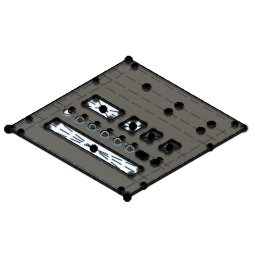
nts-1 v14 (Autodesk Fusion 360 design; units mm, degrees)
Autodesk Fusion 360 part; units mm, degrees
sketch "Sketch1" plane through (0, 0, 0) normal (0, 0, 1) x (1, 0, 0)
  line L0 (2, 0) -> (126.53, 0)
  line L1 (128.53, 2) -> (128.53, 128)
  line L2 (126.53, 130) -> (2, 130)
  line L3 (0, 128) -> (0, 2)
  line L4 (0, 70) -> (128.53, 70) construction
  line L5 (0, 46.94) -> (128.53, 46.94) construction
  line L6 (0, 92) -> (128.53, 92) construction
  line L7 (0, 20) -> (128.53, 20) construction
  line L8 (2.5, 130) -> (2.5, 0) construction
  line L9 (126.03, 130) -> (126.03, 0) construction
  circle A0 centre (71, 46.94) radius 3.55
  circle A1 centre (17, 46.94) radius 3.55
  circle A2 centre (84.5, 46.94) radius 3.55
  circle A3 centre (30.5, 46.94) radius 3.55
  circle A4 centre (111.53, 46.94) radius 3.55
  circle A5 centre (44, 46.94) radius 3.55
  circle A6 centre (57.5, 46.94) radius 3.55
  circle A7 centre (126.03, 92) radius 1.5
  circle A8 centre (2.5, 92) radius 1.5
  circle A9 centre (2.5, 20) radius 1.5
  circle A10 centre (126.03, 20) radius 1.5
  line L10 (107.73, 62.5) -> (101.33, 62.5)
  line L11 (99.03, 64.8) -> (99.03, 75.2)
  line L12 (101.33, 77.5) -> (107.73, 77.5)
  line L13 (110.03, 75.2) -> (110.03, 64.8)
  line L14 (110.03, 62.5) -> (99.03, 77.5) construction
  line L15 (99.03, 62.5) -> (110.03, 77.5) construction
  line L16 (88.03, 62.5) -> (81.33, 62.5)
  line L17 (79.03, 64.8) -> (79.03, 75.5)
  line L18 (81.03, 77.5) -> (88.03, 77.5)
  line L19 (90.03, 75.5) -> (90.03, 64.5)
  line L20 (90.03, 62.5) -> (79.03, 77.5) construction
  line L21 (79.03, 62.5) -> (90.03, 77.5) construction
  line L22 (70.03, 61.5) -> (59.03, 61.5)
  line L23 (57.03, 63.5) -> (57.03, 76.5)
  line L24 (59.03, 78.5) -> (70.03, 78.5)
  line L25 (72.03, 76.5) -> (72.03, 63.5)
  line L26 (72.03, 61.5) -> (57.03, 78.5) construction
  line L27 (57.03, 61.5) -> (72.03, 78.5) construction
  line L28 (46.53, 62) -> (18.53, 62)
  line L29 (16.53, 64) -> (16.53, 76)
  line L30 (18.53, 78) -> (46.53, 78)
  line L31 (48.53, 76) -> (48.53, 64)
  line L32 (48.53, 62) -> (16.53, 78) construction
  line L33 (16.53, 62) -> (48.53, 78) construction
  line L34 (100.23, 49.94) -> (94.83, 49.94)
  line L35 (92.53, 47.64) -> (92.53, 46.24)
  line L36 (94.83, 43.94) -> (100.23, 43.94)
  line L37 (102.53, 46.24) -> (102.53, 47.64)
  line L38 (102.53, 49.94) -> (92.53, 43.94) construction
  line L39 (92.53, 49.94) -> (102.53, 43.94) construction
  arc A11 (2, 130) -> (0, 128) centre (2, 128) ccw
  arc A12 (128.53, 128) -> (126.53, 130) centre (126.53, 128) ccw
  arc A13 (126.53, 0) -> (128.53, 2) centre (126.53, 2) ccw
  arc A14 (0, 2) -> (2, 0) centre (2, 2) ccw
  arc A15 (18.53, 78) -> (16.53, 76) centre (18.53, 76) ccw
  arc A16 (46.53, 62) -> (48.53, 64) centre (46.53, 64) ccw
  arc A17 (16.53, 64) -> (18.53, 62) centre (18.53, 64) ccw
  arc A18 (48.53, 76) -> (46.53, 78) centre (46.53, 76) ccw
  arc A19 (59.03, 78.5) -> (57.03, 76.5) centre (59.03, 76.5) ccw
  arc A20 (72.03, 76.5) -> (70.03, 78.5) centre (70.03, 76.5) ccw
  arc A21 (70.03, 61.5) -> (72.03, 63.5) centre (70.03, 63.5) ccw
  arc A22 (57.03, 63.5) -> (59.03, 61.5) centre (59.03, 63.5) ccw
  arc A23 (81.03, 77.5) -> (79.03, 75.5) centre (81.03, 75.5) ccw
  arc A24 (90.03, 75.5) -> (88.03, 77.5) centre (88.03, 75.5) ccw
  arc A25 (88.03, 62.5) -> (90.03, 64.5) centre (88.03, 64.5) ccw
  arc A26 (79.03, 64.8) -> (81.33, 62.5) centre (81.33, 64.8) ccw
  arc A27 (101.33, 77.5) -> (99.03, 75.2) centre (101.33, 75.2) ccw
  arc A28 (110.03, 75.2) -> (107.73, 77.5) centre (107.73, 75.2) ccw
  arc A29 (107.73, 62.5) -> (110.03, 64.8) centre (107.73, 64.8) ccw
  arc A30 (99.03, 64.8) -> (101.33, 62.5) centre (101.33, 64.8) ccw
  arc A31 (94.83, 49.94) -> (92.53, 47.64) centre (94.83, 47.64) ccw
  arc A32 (102.53, 47.64) -> (100.23, 49.94) centre (100.23, 47.64) ccw
  arc A33 (92.53, 46.24) -> (94.83, 43.94) centre (94.83, 46.24) ccw
  arc A34 (100.23, 43.94) -> (102.53, 46.24) centre (100.23, 46.24) ccw
  line L40 (0, 126.5) -> (128.53, 126.5) construction
  line L41 (0, 3.5) -> (128.53, 3.5) construction
  line L42 (118.53, 130) -> (118.53, 0) construction
  line L43 (10, 130) -> (10, 0) construction
  circle A35 centre (10, 126.5) radius 2
  circle A36 centre (118.53, 126.5) radius 2
  circle A37 centre (10, 3.5) radius 2
  circle A38 centre (118.53, 3.5) radius 2
  line L44 (0, 28) -> (128.53, 28) construction
  line L45 (109.765, 20.75) -> (18.765, 20.75)
  line L46 (16.765, 22.75) -> (16.765, 33.25)
  line L47 (18.765, 35.25) -> (109.765, 35.25)
  line L48 (111.765, 33.25) -> (111.765, 22.75)
  line L49 (111.765, 20.75) -> (16.765, 35.25) construction
  line L50 (16.765, 20.75) -> (111.765, 35.25) construction
  arc A39 (18.765, 35.25) -> (16.765, 33.25) centre (18.765, 33.25) ccw
  arc A40 (111.765, 33.25) -> (109.765, 35.25) centre (109.765, 33.25) ccw
  arc A41 (16.765, 22.75) -> (18.765, 20.75) centre (18.765, 22.75) ccw
  arc A42 (109.765, 20.75) -> (111.765, 22.75) centre (109.765, 22.75) ccw
  line L51 (0, 113.5) -> (128.53, 113.5) construction
  line L52 (0, 102) -> (128.53, 102) construction
  circle A43 centre (106.03, 113.5) radius 3.25
  circle A44 centre (106.03, 102) radius 3.25
  circle A45 centre (71.03, 113.5) radius 3.25
  circle A46 centre (71.03, 102) radius 3.25
  circle A47 centre (36.03, 113.5) radius 3.25
  line L53 (0, 51.84) -> (128.53, 51.84) construction
  circle A48 centre (17, 51.84) radius 0.75
  circle A49 centre (30.5, 51.84) radius 0.75
  circle A50 centre (44, 51.84) radius 0.75
  circle A51 centre (57.5, 51.84) radius 0.75
  circle A52 centre (71, 51.84) radius 0.75
  circle A53 centre (84.5, 51.84) radius 0.75
  circle A54 centre (111.53, 51.84) radius 0.75
  point P0 (128.53, 0)
  point P1 (0, 130)
  point P2 (104.53, 70)
  point P3 (84.53, 70)
  point P4 (64.53, 70)
  point P5 (32.53, 70)
  point P6 (97.53, 46.94)
  point P7 (64.265, 28)
  dimension "d1" = 128.53
  dimension "d2" = 130
  dimension "d4" = 2.5
  dimension "d5" = 2.5
  dimension "d7" = 60
  dimension "d25" = 7.1
  dimension "d26" = 7.1
  dimension "d27" = 7.1
  dimension "d28" = 7.1
  dimension "d29" = 7.1
  dimension "d30" = 7.1
  dimension "d31" = 7.1
  dimension "d32" = 17
  dimension "d33" = 13.5
  dimension "d34" = 13.5
  dimension "d35" = 13.5
  dimension "d36" = 13.5
  dimension "d37" = 13.5
  dimension "d38" = 17
  dimension "d42" = 3
  dimension "d43" = 3
  dimension "d44" = 3
  dimension "d45" = 3
  dimension "d49" = 72
  dimension "d54" = 23.06
  dimension "d55" = 22
  dimension "d56" = 11
  dimension "d57" = 15
  dimension "d58" = 24
  dimension "d59" = 11
  dimension "d60" = 15
  dimension "d61" = 20
  dimension "d62" = 15
  dimension "d63" = 17
  dimension "d64" = 20
  dimension "d65" = 32
  dimension "d66" = 16
  dimension "d67" = 32
  dimension "d68" = 10
  dimension "d69" = 6
  dimension "d70" = 14
  dimension "d75" = 2
  dimension "d76" = 2
  dimension "d77" = 2
  dimension "d78" = 2
  dimension "d79" = 2
  dimension "d80" = 2
  dimension "d81" = 2
  dimension "d82" = 2
  dimension "d83" = 2
  dimension "d84" = 2
  dimension "d85" = 2.3
  dimension "d86" = 123
  dimension "d87" = 3.5
  dimension "d89" = 4
  dimension "d90" = 4
  dimension "d91" = 4
  dimension "d92" = 4
  dimension "d93" = 10
  dimension "d94" = 10
  dimension "d99" = 42
  dimension "d100" = 95
  dimension "d101" = 14.5
  dimension "d102" = 2
  dimension "d103" = 2
  dimension "d104" = 2
  dimension "d105" = 2
  dimension "d106" = 32
  dimension "d107" = 11.5
  dimension "d110" = 6.5
  dimension "d111" = 6.5
  dimension "d112" = 6.5
  dimension "d113" = 6.5
  dimension "d117" = 35
  dimension "d118" = 20
  dimension "d121" = 6.5
  dimension "d122" = 35
  dimension "d123" = 4.9
  dimension "d126" = 1.5
  dimension "d127" = 17
  dimension "d128" = 1.5
  dimension "d129" = 1.5
  dimension "d130" = 1.5
  dimension "d131" = 1.5
  dimension "d132" = 1.5
  dimension "d133" = 1.5
  dimension "d134" = 17
  dimension "d135" = 13.5
  dimension "d136" = 13.5
  dimension "d137" = 13.5
  dimension "d138" = 13.5
  dimension "d139" = 13.5
  constraint horizontal L0
  constraint vertical L1
  constraint horizontal L2
  constraint vertical L3
  constraint coincident L3 L4.start
  constraint coincident L1 L4.end
  constraint perpendicular L1 L4
  constraint coincident L3 L5.start
  constraint perpendicular L3 L5
  constraint coincident L1 L5.end
  constraint coincident L3 L6.start
  constraint perpendicular L3 L6
  constraint coincident L1 L6.end
  constraint coincident L3 L7.start
  constraint perpendicular L3 L7
  constraint coincident L1 L7.end
  constraint coincident L2 L8.start
  constraint perpendicular L2 L8
  constraint coincident L0 L8.end
  constraint coincident L2 L9.start
  constraint perpendicular L2 L9
  constraint coincident L0 L9.end
  constraint coincident L5 A0.centre
  constraint coincident L5 A2.centre
  constraint coincident L5 A3.centre
  constraint coincident L5 A4.centre
  constraint coincident L5 A5.centre
  constraint coincident L5 A6.centre
  constraint coincident L9 A7.centre
  constraint coincident L6 A7.centre
  constraint coincident L8 A8.centre
  constraint coincident L6 A8.centre
  constraint coincident L8 A9.centre
  constraint coincident L7 A9.centre
  constraint coincident L9 A10.centre
  constraint coincident L7 A10.centre
  constraint horizontal L10
  constraint perpendicular L10 L11
  constraint parallel L10 L12
  constraint parallel L11 L13
  constraint coincident L14 P2
  constraint coincident L15 P2
  constraint coincident L4 P2
  constraint horizontal L16
  constraint perpendicular L16 L17
  constraint parallel L16 L18
  constraint parallel L17 L19
  constraint coincident L20 P3
  constraint coincident L21 P3
  constraint coincident L4 P3
  constraint horizontal L22
  constraint perpendicular L22 L23
  constraint parallel L22 L24
  constraint parallel L23 L25
  constraint coincident L26 P4
  constraint coincident L27 P4
  constraint coincident L4 P4
  constraint horizontal L28
  constraint perpendicular L28 L29
  constraint parallel L28 L30
  constraint parallel L29 L31
  constraint coincident L32 P5
  constraint coincident L33 P5
  constraint coincident L4 P5
  constraint horizontal L34
  constraint perpendicular L34 L35
  constraint parallel L34 L36
  constraint parallel L35 L37
  constraint coincident L38 P6
  constraint coincident L39 P6
  constraint coincident L5 P6
  constraint coincident P1 L2
  constraint coincident P1 L3
  constraint tangent L2 A11
  constraint tangent L3 A11
  constraint tangent L1 A12
  constraint tangent L2 A12
  constraint coincident P0 L0
  constraint coincident P0 L1
  constraint tangent L0 A13
  constraint tangent L1 A13
  constraint coincident origin L0
  constraint coincident origin L3
  constraint tangent L0 A14
  constraint tangent L3 A14
  constraint coincident L32.end L29
  constraint coincident L32.end L30
  constraint tangent L29 A15
  constraint tangent L30 A15
  constraint coincident L32.start L28
  constraint coincident L32.start L31
  constraint tangent L28 A16
  constraint tangent L31 A16
  constraint coincident L33.start L29
  constraint coincident L33.start L28
  constraint tangent L29 A17
  constraint tangent L28 A17
  constraint coincident L33.end L30
  constraint coincident L33.end L31
  constraint tangent L30 A18
  constraint tangent L31 A18
  constraint coincident L26.end L23
  constraint coincident L26.end L24
  constraint tangent L23 A19
  constraint tangent L24 A19
  constraint coincident L27.end L24
  constraint coincident L27.end L25
  constraint tangent L24 A20
  constraint tangent L25 A20
  constraint equal A19 A20
  constraint coincident L26.start L25
  constraint coincident L26.start L22
  constraint tangent L25 A21
  constraint tangent L22 A21
  constraint equal A19 A21
  constraint coincident L27.start L22
  constraint coincident L27.start L23
  constraint tangent L22 A22
  constraint tangent L23 A22
  constraint equal A19 A22
  constraint coincident L20.end L17
  constraint coincident L20.end L18
  constraint tangent L17 A23
  constraint tangent L18 A23
  constraint equal A19 A23
  constraint coincident L21.end L18
  constraint coincident L21.end L19
  constraint tangent L18 A24
  constraint tangent L19 A24
  constraint equal A19 A24
  constraint coincident L20.start L19
  constraint coincident L20.start L16
  constraint tangent L19 A25
  constraint tangent L16 A25
  constraint coincident L21.start L17
  constraint coincident L21.start L16
  constraint tangent L17 A26
  constraint tangent L16 A26
  constraint coincident L14.end L11
  constraint coincident L14.end L12
  constraint tangent L11 A27
  constraint tangent L12 A27
  constraint equal A26 A27
  constraint coincident L15.end L12
  constraint coincident L15.end L13
  constraint tangent L12 A28
  constraint tangent L13 A28
  constraint equal A26 A28
  constraint coincident L14.start L13
  constraint coincident L14.start L10
  constraint tangent L13 A29
  constraint tangent L10 A29
  constraint equal A26 A29
  constraint coincident L15.start L11
  constraint coincident L15.start L10
  constraint tangent L11 A30
  constraint tangent L10 A30
  constraint equal A26 A30
  constraint coincident L39.start L34
  constraint coincident L39.start L35
  constraint tangent L34 A31
  constraint tangent L35 A31
  constraint equal A26 A31
  constraint coincident L38.start L34
  constraint coincident L38.start L37
  constraint tangent L34 A32
  constraint tangent L37 A32
  constraint equal A26 A32
  constraint coincident L38.end L35
  constraint coincident L38.end L36
  constraint tangent L35 A33
  constraint tangent L36 A33
  constraint equal A26 A33
  constraint coincident L39.end L36
  constraint coincident L39.end L37
  constraint tangent L36 A34
  constraint tangent L37 A34
  constraint equal A26 A34
  constraint coincident L3 L40.start
  constraint perpendicular L3 L40
  constraint coincident L1 L40.end
  constraint coincident L3 L41.start
  constraint perpendicular L3 L41
  constraint coincident L1 L41.end
  constraint coincident L2 L42.start
  constraint coincident L0 L42.end
  constraint perpendicular L0 L42
  constraint coincident L2 L43.start
  constraint coincident L0 L43.end
  constraint perpendicular L0 L43
  constraint coincident L43 A35.centre
  constraint coincident L40 A35.centre
  constraint coincident L42 A36.centre
  constraint coincident L40 A36.centre
  constraint coincident L43 A37.centre
  constraint coincident L41 A37.centre
  constraint coincident L42 A38.centre
  constraint coincident L41 A38.centre
  constraint coincident L3 L44.start
  constraint perpendicular L3 L44
  constraint coincident L1 L44.end
  constraint horizontal L45
  constraint perpendicular L45 L46
  constraint parallel L45 L47
  constraint parallel L46 L48
  constraint coincident L49 P7
  constraint coincident L50 P7
  constraint midpoint L44 P7
  constraint coincident L49.end L46
  constraint coincident L49.end L47
  constraint tangent L46 A39
  constraint tangent L47 A39
  constraint coincident L50.end L47
  constraint coincident L50.end L48
  constraint tangent L47 A40
  constraint tangent L48 A40
  constraint coincident L50.start L46
  constraint coincident L50.start L45
  constraint tangent L46 A41
  constraint tangent L45 A41
  constraint coincident L49.start L48
  constraint coincident L49.start L45
  constraint tangent L48 A42
  constraint tangent L45 A42
  constraint coincident L3 L51.start
  constraint perpendicular L3 L51
  constraint coincident L1 L51.end
  constraint coincident L3 L52.start
  constraint perpendicular L3 L52
  constraint coincident L1 L52.end
  constraint coincident L51 A43.centre
  constraint coincident L52 A44.centre
  constraint coincident L51 A45.centre
  constraint coincident L52 A46.centre
  constraint vertical A45.centre A46.centre
  constraint vertical A43.centre A44.centre
  constraint coincident L51 A47.centre
  constraint coincident L3 L53.start
  constraint perpendicular L3 L53
  constraint coincident L1 L53.end
  constraint coincident L53 A48.centre
  constraint coincident L53 A49.centre
  constraint coincident L53 A50.centre
  constraint coincident L53 A51.centre
  constraint coincident L53 A52.centre
  constraint coincident L53 A53.centre
  constraint coincident L53 A54.centre
  measures "d1" distance of origin P0
  measures "d2" distance of origin P1
  measures "d4" distance of L3 L8
  measures "d5" distance of L1 L9
  measures "d7" distance of L2 L4
  measures "d25" diameter of A0
  measures "d26" diameter of A1
  measures "d27" diameter of A2
  measures "d28" diameter of A3
  measures "d29" diameter of A4
  measures "d30" diameter of A5
  measures "d31" diameter of A6
  measures "d32" distance of L3 A1.centre
  measures "d33" distance of A1.centre A3.centre
  measures "d34" distance of A3.centre A5.centre
  measures "d35" distance of A5.centre A6.centre
  measures "d36" distance of A0.centre A6.centre
  measures "d37" distance of A0.centre A2.centre
  measures "d38" distance of L1 A4.centre
  measures "d42" diameter of A7
  measures "d43" diameter of A8
  measures "d44" diameter of A9
  measures "d45" diameter of A10
  measures "d49" distance of A7.centre A10.centre
  measures "d54" distance of L4 L5
  measures "d55" distance of L4 L6
  measures "d56" distance of L14.end L15.end
  measures "d57" distance of L15.start L14.end
  measures "d58" distance of L4.end P2
  measures "d59" distance of L20.end L21.end
  measures "d60" distance of L21.start L20.end
  measures "d61" distance of P2 P3
  measures "d62" distance of L26.end L27.end
  measures "d63" distance of L27.start L26.end
  measures "d64" distance of P3 P4
  measures "d65" distance of L32.end L33.end
  measures "d66" distance of L33.start L32.end
  measures "d67" distance of P4 P5
  measures "d68" distance of L38.end L39.end
  measures "d69" distance of L39.start L38.end
  measures "d70" distance of A4.centre P6
  measures "d75" radius of A11
  measures "d76" radius of A12
  measures "d77" radius of A13
  measures "d78" radius of A14
  measures "d79" radius of A15
  measures "d80" radius of A16
  measures "d81" radius of A17
  measures "d82" radius of A18
  measures "d83" radius of A19
  measures "d84" radius of A25
  measures "d85" radius of A26
  measures "d86" distance of L40 L41
  measures "d87" distance of L2 L40
  measures "d89" diameter of A35
  measures "d90" diameter of A36
  measures "d91" diameter of A37
  measures "d92" diameter of A38
  measures "d93" distance of L3 L43
  measures "d94" distance of L1 L42
  measures "d99" distance of L4 L44
  measures "d100" distance of L49.end L50.end
  measures "d101" distance of L50.start L49.end
  measures "d102" radius of A39
  measures "d103" radius of A40
  measures "d104" radius of A41
  measures "d105" radius of A42
  measures "d106" distance of L4 L52
  measures "d107" distance of L51 L52
  measures "d110" diameter of A43
  measures "d111" diameter of A44
  measures "d112" diameter of A45
  measures "d113" diameter of A46
  measures "d117" distance of A44.centre A46.centre
  measures "d118" distance of L9 A43.centre
  measures "d121" diameter of A47
  measures "d122" distance of A45.centre A47.centre
  measures "d123" distance of L5 L53
  measures "d126" diameter of A48
  measures "d127" distance of L53.start A48.centre
  measures "d128" diameter of A49
  measures "d129" diameter of A50
  measures "d130" diameter of A51
  measures "d131" diameter of A52
  measures "d132" diameter of A53
  measures "d133" diameter of A54
  measures "d134" distance of L1 A54.centre
  measures "d135" distance of A48.centre A49.centre
  measures "d136" distance of A49.centre A50.centre
  measures "d137" distance of A50.centre A51.centre
  measures "d138" distance of A51.centre A52.centre
  measures "d139" distance of A52.centre A53.centre
extrude "Extrude5" add sketch "Sketch1" along normal blind 1.5
equation "d7 = Offset_from_top"
equation "d25 = button_size"
equation "d26 = button_size"
equation "d27 = button_size"
equation "d28 = button_size"
equation "d29 = button_size"
equation "d30 = button_size"
equation "d31 = button_size"
equation "d33 = button_spacing"
equation "d34 = button_spacing"
equation "d35 = button_spacing"
equation "d36 = button_spacing"
equation "d37 = button_spacing"
equation "d42 = mount_hole"
equation "d43 = mount_hole"
equation "d44 = mount_hole"
equation "d45 = mount_hole"
equation "button_spacing = 13.5 mm"
equation "button_size = 7.1 mm"
equation "euro_screw_hole = 4 mm"
equation "d89 = euro_screw_hole"
equation "d90 = euro_screw_hole"
equation "d91 = euro_screw_hole"
equation "d92 = euro_screw_hole"
equation "mount_hole = 3 mm"
equation "Offset_from_top = 60 mm"
equation "audio_jack_hole = 6.5 mm"
equation "d110 = audio_jack_hole"
equation "d111 = audio_jack_hole"
equation "d112 = audio_jack_hole"
equation "d113 = audio_jack_hole"
equation "d121 = audio_jack_hole"
equation "led = 1.5 mm"
equation "d126 = led"
equation "d128 = led"
equation "d129 = led"
equation "d130 = led"
equation "d131 = led"
equation "d132 = led"
equation "d133 = led"
equation "d135 = button_spacing"
equation "d136 = button_spacing"
equation "d137 = button_spacing"
equation "d138 = button_spacing"
equation "d139 = button_spacing"
